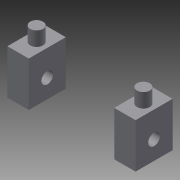
# Autodesk Inventor part: FretterMountBottom
Saved by Autodesk Inventor 2015 (Build 190159000, 159)
## iProperties
Created: 2016-05-03
Part Number: FretterMountBottom
Material: Generic
Document SubType Name: Modeling
Designer: Hatch
Density: 1 g/cm^3
Appearance: Default
Author: Hatch
Autodesk Inventor part; units mm, degrees
ref_plane "YZ Plane" through (0, 0, 0) normal (1, 0, 0) x (0, 1, 0)
ref_plane "XZ Plane" through (0, 0, 0) normal (0, 1, 0) x (-1, 0, 0)
ref_plane "XY Plane" through (0, 0, 0) normal (0, 0, 1) x (1, 0, 0)
sketch "Sketch1" plane through (0, 0, 0) normal (0, 1, 0) x (-1, 0, 0)
  line L0 (0, 0) -> (0, -14)
  circle A0 centre (0, -7) radius 8.25
  circle A1 centre (0, -7) radius 10.5
  dimension "d0" = 14
  dimension "d1" = 16.5
  dimension "d2" = 21
  constraints: 2 centre point, 2 end point, 1 coincident, 1 midpoint, 1 vertical
  measures "d0" distance of L0.start L0.end
  measures "d1" diameter of A0
  measures "d2" diameter of A1
extrude "Extrusion1" add sketch "Sketch1" along normal blind 6
sketch "Sketch2" plane through (0, 6, -7) normal (0, 1, 0) x (1, 0, 0)
  line L0 (10.5, -10.5) -> (-10.5, -10.5)
  line L1 (-10.5, -10.5) -> (-10.5, 10.5)
  line L2 (-10.5, 10.5) -> (10.5, 10.5)
  line L3 (10.5, 10.5) -> (10.5, -10.5)
  line L4 (10.5, -10.5) -> (-10.5, 10.5) construction
  line L5 (-10.5, -10.5) -> (10.5, 10.5) construction
  circle A0 centre (0, 0) radius 10.5
  point P0 (0, -7)
  constraints: 12 end point, 2 midpoint, 2 parallel, 1 centre point, 1 coincident, 1 horizontal, 1 perpendicular
extrude "Extrusion2" add sketch "Sketch2" against normal blind 6 contours L0 A0 L3 | L0 L1 A0 | A0 L2 L3 | L1 L2 A0
sketch "Sketch4" plane through (0, 6, 0) normal (0, 1, 0) x (1, 0, 0)
  circle A0 centre (0, 7) radius 8.25 projected
  line L0 (0, 7) -> (0, -0.25)
  line L1 (0, -0.25) -> (-3.937, -0.25)
  line L2 (3.937, -0.25) -> (-3.937, -0.25)
  point P0 (0, 0)
  dimension "d14" = 7.25
  constraints: 6 end point, 2 point on circle, 1 collinear, 1 perpendicular, 1 point on line, 1 vertical
  measures "d14" distance of L0.start L0.end
extrude "Extrusion4" add sketch "Sketch4" against normal blind 6 contours L1 L2 A0 picked at (1.9893, -0.4987)
pattern_circular "Circular Pattern2" count 6 over 360 about axis through (0, 0, -7) along (0, 1, 0) of "Extrusion4"
sketch "Sketch5" plane through (0, 6, 0) normal (0, 1, 0) x (1, 0, 0)
  line L0 (-4.3102, -0.0345) -> (-8.2472, 6.7845) projected
  line L1 (-6.2787, 3.375) -> (6.2787, 10.625)
  line L2 (4.3102, 14.0345) -> (8.2472, 7.2155) projected
  line L3 (8.2472, 6.7845) -> (4.3102, -0.0345) projected
  line L4 (6.2787, 3.375) -> (-6.2787, 10.625)
  line L5 (-4.3102, 14.0345) -> (-8.2472, 7.2155) projected
  line L6 (3.937, 14.25) -> (-3.937, 14.25) projected
  line L7 (0, 14.25) -> (0, -0.25)
  line L8 (3.937, -0.25) -> (-3.937, -0.25) projected
  circle A0 centre (0, 7) radius 9.625
  line L9 (12.5, 19.5) -> (-12.5, 19.5)
  line L10 (-12.5, 19.5) -> (-12.5, -5.5)
  line L11 (-12.5, -5.5) -> (12.5, -5.5)
  line L12 (12.5, -5.5) -> (12.5, 19.5)
  line L13 (12.5, 19.5) -> (-12.5, -5.5) construction
  line L14 (-12.5, 19.5) -> (12.5, -5.5) construction
  point P0 (0, 0)
  dimension "d20" = 19.25
  dimension "d21" = 25
  dimension "d22" = 25
  constraints: 18 end point, 9 midpoint, 2 parallel, 1 centre point, 1 horizontal, 1 perpendicular
  measures "d20" diameter of A0
  measures "d21" distance of L11.end L10.end
  measures "d22" distance of L10.end L9.end
extrude "Extrusion5" add sketch "Sketch5" along normal blind 20
sketch "Sketch6" plane through (0, 6, 0) normal (0, -1, 0) x (1, 0, 0)
  line L0 (-10.5, -17.5) -> (10.5, -17.5)
  line L1 (10.5, -17.5) -> (10.5, 3.5)
  line L2 (10.5, 3.5) -> (-10.5, 3.5)
  line L3 (-10.5, 3.5) -> (-10.5, -17.5)
  circle A0 centre (0, -7) radius 9.625 projected
  line L4 (-10.5, -17.5) -> (10.5, 3.5) construction
  line L5 (10.5, -17.5) -> (-10.5, 3.5) construction
  line L6 (-12.5, -19.5) -> (12.5, -19.5)
  line L7 (12.5, -19.5) -> (12.5, 5.5)
  line L8 (12.5, 5.5) -> (-12.5, 5.5)
  line L9 (-12.5, 5.5) -> (-12.5, -19.5)
  line L10 (-12.5, -19.5) -> (12.5, 5.5) construction
  line L11 (12.5, -19.5) -> (-12.5, 5.5) construction
  point P0 (0, 0)
  constraints: 24 end point, 4 midpoint, 4 parallel, 2 horizontal, 2 perpendicular
extrude "Extrusion6" add sketch "Sketch6" along normal blind 6 contours L9 L8 L7 L6
sketch "Sketch8" plane through (-12.5, 26, 5.5) normal (0, 0, 1) x (1, 0, 0)
  line L0 (0, 0) -> (25, 0)
  line L1 (0, 0) -> (-17.5, 0)
  line L2 (25, 0) -> (42.5, 0)
  line L3 (0, 0) -> (-17.5, 0)
  line L4 (-17.5, 0) -> (-17.5, -26)
  line L5 (-17.5, -26) -> (0, -26)
  line L6 (0, -26) -> (0, 0)
  line L7 (25, 0) -> (42.5, 0)
  line L8 (42.5, 0) -> (42.5, -26)
  line L9 (42.5, -26) -> (25, -26)
  line L10 (25, -26) -> (25, 0)
  point P0 (12.5, -26)
  dimension "d27" = 17.5
  dimension "d28" = 17.5
  constraints: 22 end point, 5 horizontal, 4 parallel, 2 perpendicular, 1 point on line
  measures "d27" distance of L0.start L1.end
  measures "d28" distance of L0.end L2.end
extrude "Extrusion7" add sketch "Sketch8" against normal blind 25
sketch "Sketch9" plane through (-30, 0, 5.5) normal (0, 0, 1) x (1, 0, 0)
  line L0 (0, 26) -> (-15, 26)
  line L1 (-15, 26) -> (-15, 0)
  line L2 (-15, 0) -> (0, 0)
  line L3 (0, 0) -> (0, 26)
  line L4 (60, 26) -> (75, 26)
  line L5 (75, 26) -> (75, 0)
  line L6 (75, 0) -> (60, 0)
  line L7 (60, 0) -> (60, 26)
  point P0 (30, 0)
  dimension "d31" = 15
  dimension "d32" = 15
  constraints: 16 end point, 4 parallel, 2 horizontal, 2 perpendicular, 1 point on line
  measures "d31" distance of L2.end L1.end
  measures "d32" distance of L5.end L6.end
extrude "Extrusion8" add sketch "Sketch9" against normal blind 61.25
sketch "Sketch10" plane through (-45, 0, 5.5) normal (-1, 0, 0) x (0, 0, 1)
  line L0 (-61.25, 0) -> (-61.25, 26) projected
  line L1 (-61.25, 13) -> (-35, 13)
  circle A0 centre (-48.125, 13) radius 4.125
  point P0 (-5.5, 0)
  dimension "d35" = 26.25
  dimension "d36" = 8.25
  constraints: 2 end point, 2 midpoint, 1 centre point, 1 horizontal
  measures "d35" distance of L1.start L1.end
  measures "d36" diameter of A0
extrude "Extrusion9" cut sketch "Sketch10" against normal through all
sketch "Sketch11" plane through (0, 26, 0) normal (0, 1, 0) x (1, 0, 0)
  line L0 (30, 19.5) -> (30, 24.5)
  line L1 (30, 19.5) -> (30, 55.75) projected
  line L2 (30, 19.5) -> (25, 19.5)
  line L3 (25, 19.5) -> (30, 24.5)
  line L4 (-30, 19.5) -> (-30, 24.5)
  line L5 (-30, 19.5) -> (-30, 55.75) projected
  line L6 (-30, 19.5) -> (-25, 19.5)
  line L7 (30, 19.5) -> (-30, 19.5) projected
  line L8 (-25, 19.5) -> (-30, 24.5)
  point P0 (0, 0)
  dimension "d39" = 5
  dimension "d40" = 5
  dimension "d41" = 5
  dimension "d42" = 5
  constraints: 12 end point, 3 point on line, 1 horizontal
  measures "d39" distance of L0.start L0.end
  measures "d40" distance of L0.start L2.end
  measures "d41" distance of L4.start L4.end
  measures "d42" distance of L4.start L6.end
extrude "Extrusion10" add sketch "Sketch11" against normal blind 26
sketch "Sketch12" plane through (0, 26, 0) normal (0, 1, 0) x (1, 0, 0)
  line L0 (-45, -5.5) -> (-45, 55.75) projected
  line L1 (45, -5.5) -> (-45, -5.5)
  line L2 (-45, -5.5) -> (-45, 24.5)
  line L3 (-45, 24.5) -> (45, 24.5)
  line L4 (45, 24.5) -> (45, -5.5)
  point P0 (0, 0)
  constraints: 8 end point, 2 parallel, 1 horizontal, 1 perpendicular, 1 point on line
extrude "Extrusion11" cut sketch "Sketch12" against normal through all
sketch "Sketch13" plane through (-45, 26, -24.5) normal (0, 0, 1) x (1, 0, 0)
  circle A0 centre (7.5, -13) radius 4.5
  circle A1 centre (82.5, -13) radius 4.5
  point P0 (45, -26)
  dimension "d47" = 9
  dimension "d48" = 9
  constraints: 2 centre point
  measures "d47" diameter of A0
  measures "d48" diameter of A1
extrude "Extrusion12" add sketch "Sketch13" along normal blind 10
body "Solid1"
